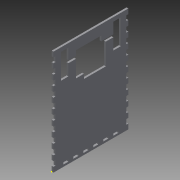
# Autodesk Inventor part: onderplaat
Saved by Autodesk Inventor 2015 (Build 190159000, 159)
## iProperties
Created: 2016-03-10
Part Number: onderplaat
Material: Generic
Document SubType Name: Modeling
Designer: david
Density: 1 g/cm^3
Appearance: Default
Author: david
Autodesk Inventor part; units mm, degrees
ref_plane "YZ Plane" through (0, 0, 0) normal (1, 0, 0) x (0, 1, 0)
ref_plane "XZ Plane" through (0, 0, 0) normal (0, 1, 0) x (-1, 0, 0)
ref_plane "XY Plane" through (0, 0, 0) normal (0, 0, 1) x (1, 0, 0)
sketch "Sketch1" plane through (0, 0, 0) normal (1, 0, 0) x (0, 1, 0)
  line L0 (0, 0) -> (150, 0)
  line L1 (150, 0) -> (150, 210)
  line L2 (150, 210) -> (0, 210)
  line L3 (0, 210) -> (0, 0)
  line L4 (105, 190) -> (45, 190)
  line L5 (45, 190) -> (45, 132)
  line L6 (45, 132) -> (105, 132)
  line L7 (105, 132) -> (105, 190)
  line L8 (105, 190) -> (96, 190)
  line L9 (96, 190) -> (96, 170)
  line L10 (96, 170) -> (105, 170)
  line L11 (105, 170) -> (105, 190)
  line L12 (45, 141) -> (61, 141)
  line L13 (61, 141) -> (61, 132)
  line L14 (61, 132) -> (45, 132)
  line L15 (45, 132) -> (45, 141)
  line L16 (105, 190) -> (96, 190)
  line L17 (96, 190) -> (96, 180)
  line L18 (96, 180) -> (105, 180)
  line L19 (105, 180) -> (105, 190)
  line L20 (105, 180) -> (135, 180)
  line L21 (135, 180) -> (135, 175)
  line L22 (135, 175) -> (105, 175)
  line L23 (105, 175) -> (105, 180)
  line L24 (135, 202) -> (120, 202)
  line L25 (120, 202) -> (120, 152)
  line L26 (120, 152) -> (135, 152)
  line L27 (135, 152) -> (135, 202)
  line L28 (105, 180) -> (26.723, 180)
  line L29 (26.723, 180) -> (26.723, 175)
  line L30 (26.723, 175) -> (105, 175)
  line L31 (105, 175) -> (105, 180)
  line L32 (45, 180) -> (15, 180)
  line L33 (15, 180) -> (15, 175)
  line L34 (15, 175) -> (45, 175)
  line L35 (45, 175) -> (45, 180)
  line L36 (30, 202) -> (15, 202)
  line L37 (15, 202) -> (15, 152)
  line L38 (15, 152) -> (30, 152)
  line L39 (30, 152) -> (30, 202)
  line L40 (150, 10) -> (146, 10)
  line L41 (146, 10) -> (146, 20)
  line L42 (146, 20) -> (150, 20)
  line L43 (150, 20) -> (150, 10)
  line L44 (4, 10) -> (0, 10)
  line L45 (0, 10) -> (0, 20)
  line L46 (0, 20) -> (4, 20)
  line L47 (4, 20) -> (4, 10)
  line L48 (150, 30) -> (146, 30)
  line L49 (146, 30) -> (146, 40)
  line L50 (146, 40) -> (150, 40)
  line L51 (150, 40) -> (150, 30)
  line L52 (150, 50) -> (146, 50)
  line L53 (146, 50) -> (146, 60)
  line L54 (146, 60) -> (150, 60)
  line L55 (150, 60) -> (150, 50)
  line L56 (150, 70) -> (146, 70)
  line L57 (146, 70) -> (146, 80)
  line L58 (146, 80) -> (150, 80)
  line L59 (150, 80) -> (150, 70)
  line L60 (150, 90) -> (146, 90)
  line L61 (146, 90) -> (146, 100)
  line L62 (146, 100) -> (150, 100)
  line L63 (150, 100) -> (150, 90)
  line L64 (150, 110) -> (146, 110)
  line L65 (146, 110) -> (146, 120)
  line L66 (146, 120) -> (150, 120)
  line L67 (150, 120) -> (150, 110)
  line L68 (150, 130) -> (146, 130)
  line L69 (146, 130) -> (146, 140)
  line L70 (146, 140) -> (150, 140)
  line L71 (150, 140) -> (150, 130)
  line L72 (150, 150) -> (146, 150)
  line L73 (146, 150) -> (146, 160)
  line L74 (146, 160) -> (150, 160)
  line L75 (150, 160) -> (150, 150)
  line L76 (150, 170) -> (146, 170)
  line L77 (146, 170) -> (146, 180)
  line L78 (146, 180) -> (150, 180)
  line L79 (150, 180) -> (150, 170)
  line L80 (150, 190) -> (146, 190)
  line L81 (146, 190) -> (146, 200)
  line L82 (146, 200) -> (150, 200)
  line L83 (150, 200) -> (150, 190)
  line L84 (4, 30) -> (0, 30)
  line L85 (0, 30) -> (0, 40)
  line L86 (0, 40) -> (4, 40)
  line L87 (4, 40) -> (4, 30)
  line L88 (4, 50) -> (0, 50)
  line L89 (0, 50) -> (0, 60)
  line L90 (0, 60) -> (4, 60)
  line L91 (4, 60) -> (4, 50)
  line L92 (4, 70) -> (0, 70)
  line L93 (0, 70) -> (0, 80)
  line L94 (0, 80) -> (4, 80)
  line L95 (4, 80) -> (4, 70)
  line L96 (4, 90) -> (0, 90)
  line L97 (0, 90) -> (0, 100)
  line L98 (0, 100) -> (4, 100)
  line L99 (4, 100) -> (4, 90)
  line L100 (4, 110) -> (0, 110)
  line L101 (0, 110) -> (0, 120)
  line L102 (0, 120) -> (4, 120)
  line L103 (4, 120) -> (4, 110)
  line L104 (4, 130) -> (0, 130)
  line L105 (0, 130) -> (0, 140)
  line L106 (0, 140) -> (4, 140)
  line L107 (4, 140) -> (4, 130)
  line L108 (4, 150) -> (0, 150)
  line L109 (0, 150) -> (0, 160)
  line L110 (0, 160) -> (4, 160)
  line L111 (4, 160) -> (4, 150)
  line L112 (4, 170) -> (0, 170)
  line L113 (0, 170) -> (0, 180)
  line L114 (0, 180) -> (4, 180)
  line L115 (4, 180) -> (4, 170)
  line L116 (4, 190) -> (0, 190)
  line L117 (0, 190) -> (0, 200)
  line L118 (0, 200) -> (4, 200)
  line L119 (4, 200) -> (4, 190)
  line L120 (126, 170) -> (126, 180)
  line L121 (106, 170) -> (106, 180)
  line L122 (86, 170) -> (86, 180)
  line L123 (66, 170) -> (66, 180)
  line L124 (46, 170) -> (46, 180)
  line L125 (26, 170) -> (26, 180)
  line L126 (30, 8) -> (20, 8)
  line L127 (20, 8) -> (20, 4)
  line L128 (20, 4) -> (30, 4)
  line L129 (30, 4) -> (30, 8)
  line L130 (50, 8) -> (40, 8)
  line L131 (40, 8) -> (40, 4)
  line L132 (40, 4) -> (50, 4)
  line L133 (50, 4) -> (50, 8)
  line L134 (70, 8) -> (60, 8)
  line L135 (60, 8) -> (60, 4)
  line L136 (60, 4) -> (70, 4)
  line L137 (70, 4) -> (70, 8)
  line L138 (90, 8) -> (80, 8)
  line L139 (80, 8) -> (80, 4)
  line L140 (80, 4) -> (90, 4)
  line L141 (90, 4) -> (90, 8)
  line L142 (110, 8) -> (100, 8)
  line L143 (100, 8) -> (100, 4)
  line L144 (100, 4) -> (110, 4)
  line L145 (110, 4) -> (110, 8)
  line L146 (130, 8) -> (120, 8)
  line L147 (120, 8) -> (120, 4)
  line L148 (120, 4) -> (130, 4)
  line L149 (130, 4) -> (130, 8)
  dimension "d0" = 150
  dimension "d1" = 210
  dimension "d2" = 60
  dimension "d3" = 45
  dimension "d4" = 20
  dimension "d5" = 58
  dimension "d6" = 20
  dimension "d7" = 9
  dimension "d8" = 16
  dimension "d9" = 9
  dimension "d10" = 30
  dimension "d11" = 5
  dimension "d12" = 15
  dimension "d13" = 50
  dimension "d14" = 22
  dimension "d15" = 30
  dimension "d16" = 5
  dimension "d17" = 15
  dimension "d18" = 50
  dimension "d19" = 15
  dimension "d20" = 0
  dimension "d25" = 4
  dimension "d26" = 10
  dimension "d27" = 10
  dimension "d28" = 4
  dimension "d29" = 10
  dimension "d30" = 10
  dimension "d35" = 20
  dimension "d42" = 20
  dimension "d49" = 20
  dimension "d54" = 22
  dimension "d57" = 4
  dimension "d58" = 10
  dimension "d59" = 20
  dimension "d60" = 4
  dimension "d63" = 20
  constraints: 300 end point, 26 parallel, 14 horizontal, 13 perpendicular, 6 point on line, 3 collinear, 2 vertical, 1 midpoint, 181 other
  measures "d0" distance of L0.start L0.end
  measures "d1" distance of L2.end L0.start
  measures "d2" distance of L5.end L6.end
  measures "d3" distance between parallel lines of L1 L7
  measures "d4" distance between parallel lines of L2 L4
  measures "d5" distance of L4.end L5.end
  measures "d6" distance of L8.end L9.end
  measures "d7" distance of L9.end L10.end
  measures "d8" distance of L12.start L12.end
  measures "d9" distance of L12.end L13.end
  measures "d10" distance of L21.end L22.end
  measures "d11" distance of L20.end L21.end
  measures "d12" distance of L25.end L26.end
  measures "d13" distance of L24.end L25.end
  measures "d14" distance between parallel lines of L20 L24
  measures "d15" distance of L33.end L34.end
  measures "d16" distance of L32.end L33.end
  measures "d17" distance of L37.end L38.end
  measures "d18" distance of L36.end L37.end
  measures "d19" distance between parallel lines of L3 L37
  measures "d20" distance between parallel lines of L21 L27
  measures "d25" distance between parallel lines of L41 L1
  measures "d26" distance between parallel lines of L0 L40
  measures "d27" distance between parallel lines of L40 L42
  measures "d28" distance between parallel lines of L3 L47
  measures "d29" distance between parallel lines of L44 L0
  measures "d30" distance between parallel lines of L44 L46
  measures "d35" distance of L41.end L50.start
  measures "d42" distance of L46.end L87.start
  measures "d49" distance of L77.start L120.start
  measures "d54" distance between parallel lines of L32 L36
  measures "d57" distance of L128.end L126.start
  measures "d58" distance of L126.start L126.end
  measures "d59" distance between parallel lines of L3 L127
  measures "d60" distance between parallel lines of L0 L128
  measures "d63" distance of L126.end L131.start
sketch "Sketch2" plane through (0, 0, 0) normal (1, 0, 0) x (0, 1, 0)
  point P0 (0, 0)
extrude "Extrusion3" add sketch "Sketch1" along normal blind 3.6 contours L3 L44 L47 L46 L84 L87 L86 L88 L91 L90 L92 L95 L94 L96 L99 L98 L100 L103 L102 L104 L107 L106 L108 L111 L110 L112 L115 L114 L116 L119 L118 L2 L1 L82 L81 L80 L78 L77 L76 L74 L73 L72 L70 L69 L68 L66 L65 L64 L62 L61 L60 L58 L57 L56 L54 L53 L52 L50 L49 L48 L42 L41 L40 L0 | L7 L18 L9 L4 | L12 L13 L6 L5
body "Solid3"
